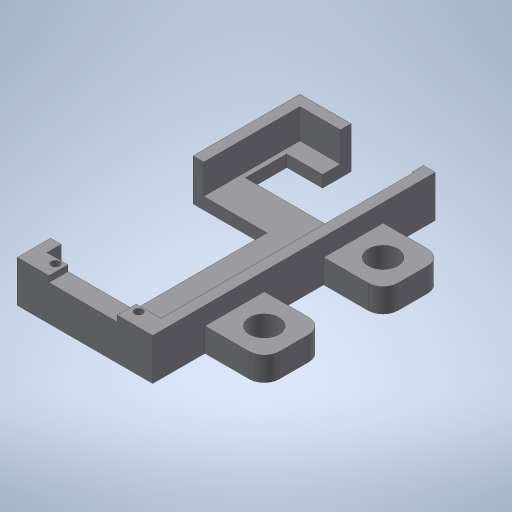
# Autodesk Inventor part: esp32-rev-tft-back-largeEncoderConn
Saved by Autodesk Inventor 2023.4 (Build 274418000, 418)
## iProperties
RuleStatus: InUse
Created: 2023-11-01
Part Number: esp32-rev-tft-back-largeEncoderConn
Project: COMMON
Material: Generic
Catalog Web Link: https://www.janelia.org/
Vendor: HHMI: JRC - jET
Document SubType Name: Modeling
Designer: sawtelles
Density: 1 g/cm^3
Appearance: Default
AfterDocSave0: file://Part Number Cleaner
LAB/DEPT: COMMON
REQUESTING SCIENTIST: COMMON
DESIGN DEPARTMENT: HHMI: JRC - jET
ALTERED ITEM PART NUMBER: N/A
ALTERED ITEM VENDOR: N/A
ALTERED ITEM DESCRIPTION: N/A
DocNumber: esp32-rev-tft=bezel
Folder: .
VDS_Category: Engineering
Title: Standard
Author: sawtelles
Revision Number: 0
Autodesk Inventor part; units mm, degrees
ref_plane "YZ Plane" through (0, 0, 0) normal (1, 0, 0) x (0, 1, 0)
ref_plane "XZ Plane" through (0, 0, 0) normal (0, 1, 0) x (-1, 0, 0)
ref_plane "XY Plane" through (0, 0, 0) normal (0, 0, 1) x (1, 0, 0)
sketch "Sketch1" plane through (0, 0, 0) normal (0, 1, 0) x (-1, 0, 0)
  line L0 (0, 0) -> (23.876, 0) construction
  line L1 (23.876, 0) -> (23.876, -71.882) construction
  line L2 (23.876, -71.882) -> (0, -71.882) construction
  line L3 (0, -71.882) -> (0, 0) construction
  line L4 (-0.254, 0.254) -> (24.13, 0.254)
  line L5 (24.13, 0.254) -> (24.13, -72.136)
  line L6 (24.13, -72.136) -> (-0.254, -72.136)
  line L7 (-0.254, -72.136) -> (-0.254, 0.254)
  circle A0 centre (5.2832, -21.971) radius 2.921
  circle A1 centre (12.2682, -21.971) radius 2.921
  circle A2 centre (19.2532, -21.971) radius 2.921
  circle A3 centre (12.2682, -58.801) radius 2.921
  circle A4 centre (21.1582, -16.891) radius 0.889
  circle A5 centre (3.3782, -16.891) radius 0.889
  circle A6 centre (21.8694, -62.611) radius 1.27
  circle A7 centre (2.7432, -62.611) radius 1.27
  line L8 (4.572, -26.416) -> (20.066, -26.416)
  line L9 (20.066, -26.416) -> (20.066, -53.848)
  line L10 (20.066, -53.848) -> (4.572, -53.848)
  line L11 (4.572, -53.848) -> (4.572, -26.416)
  dimension "d0" = 23.876
  dimension "d1" = 71.882
  dimension "d2" = 24.384
  dimension "d3" = 72.39
  dimension "d4" = 5.842
  dimension "d5" = 5.842
  dimension "d6" = 5.842
  dimension "d7" = 5.842
  dimension "d8" = 1.778
  dimension "d9" = 1.778
  dimension "d10" = 2.54
  dimension "d11" = 2.54
  dimension "d12" = 15.494
  dimension "d13" = 27.432
  dimension "d14" = 26.416
  constraints: 24 end point, 8 centre point, 6 parallel, 3 horizontal, 3 perpendicular
  measures "d0" distance of L1.end L2.end
  measures "d1" distance of L0.end L1.end
  measures "d2" distance of L5.end L6.end
  measures "d3" distance of L4.end L5.end
  measures "d4" diameter of A0
  measures "d5" diameter of A1
  measures "d6" diameter of A2
  measures "d7" diameter of A3
  measures "d8" diameter of A4
  measures "d9" diameter of A5
  measures "d10" diameter of A6
  measures "d11" diameter of A7
  measures "d12" distance of L9.end L10.end
  measures "d13" distance of L8.end L9.end
  measures "d14" distance from line of L0 L8.start
extrude "Extrusion1" add sketch "Sketch1" along normal blind 2.032
chamfer "Chamfer1" distance 0.762 angle 45 4 edges at (-16.3322, 2.032, -21.971) (-9.3472, 2.032, -21.971) (-2.3622, 2.032, -21.971) (-9.3472, 2.032, -58.801)
sketch "Sketch2" plane through (0, 0, 0) normal (0, -1, 0) x (1, 0, 0)
  line L0 (-24.13, -72.136) -> (-24.13, 0.254) projected
  line L1 (0.254, -72.136) -> (-24.13, -72.136)
  line L2 (-24.13, -72.136) -> (-24.13, -62.484)
  line L3 (-24.13, -62.484) -> (0.254, -62.484)
  line L4 (0.254, -62.484) -> (0.254, -72.136)
  line L5 (0.254, 0.254) -> (-24.13, 0.254)
  line L6 (-24.13, 0.254) -> (-24.13, -18.034)
  line L7 (-24.13, -18.034) -> (0.254, -18.034)
  line L8 (0.254, -18.034) -> (0.254, 0.254)
  circle A0 centre (-19.2532, -21.971) radius 2.921 projected
  circle A1 centre (-19.2532, -21.971) radius 2.54
  circle A2 centre (-12.1916, -21.971) radius 2.54
  circle A3 centre (-5.2239, -21.971) radius 2.54
  circle A4 centre (-12.2682, -58.801) radius 2.921 projected
  circle A5 centre (-12.2682, -58.801) radius 2.54
  point P0 (0, 0)
  point P1 (-24.13, 0.254)
  dimension "d20" = 9.652
  dimension "d21" = 18.288
  dimension "d26" = 5.08
  dimension "d27" = 5.08
  dimension "d28" = 5.08
  dimension "d29" = 5.08
  constraints: 16 end point, 4 centre point, 4 parallel, 2 coincident, 2 horizontal, 2 perpendicular, 2 point on line
  measures "d20" distance of L1.end L2.end
  measures "d21" distance of L6.end L5.end
  measures "d26" diameter of A1
  measures "d27" diameter of A2
  measures "d28" diameter of A3
  measures "d29" diameter of A5
extrude "Extrusion2" add sketch "Sketch2" along normal blind 2.032 contours L0 L3 L4 L1 | L0 L5 L8 L7
sketch "Sketch3" plane through (0, 2.032, 0) normal (0, 1, 0) x (1, 0, 0)
  circle A0 centre (-21.1582, 16.891) radius 0.889 projected
  circle A1 centre (-3.3782, 16.891) radius 0.889 projected
  circle A2 centre (-21.8694, 62.611) radius 1.27 projected
  circle A3 centre (-2.7432, 62.611) radius 1.27 projected
  point P0 (0, 0)
extrude "Extrusion3" cut sketch "Sketch3" against normal through all
sketch "Sketch4" plane through (0, 0, 0) normal (0, -1, 0) x (1, 0, 0)
  circle A0 centre (-19.2532, -21.971) radius 2.921 projected
  circle A1 centre (-19.2532, -21.971) radius 2.54
  circle A2 centre (-12.2682, -21.971) radius 2.921 projected
  circle A3 centre (-12.2682, -21.971) radius 2.54
  circle A4 centre (-5.2832, -21.971) radius 2.921 projected
  circle A5 centre (-5.2832, -21.971) radius 2.54
  circle A6 centre (-12.2682, -58.801) radius 2.921 projected
  circle A7 centre (-12.2682, -58.801) radius 2.54
  point P0 (0, 0)
  dimension "d30" = 5.08
  dimension "d31" = 5.08
  dimension "d32" = 5.08
  dimension "d33" = 5.08
  constraints: 4 centre point, 4 coincident
  measures "d30" diameter of A1
  measures "d31" diameter of A3
  measures "d32" diameter of A5
  measures "d33" diameter of A7
extrude "Extrusion4" [suppressed]
sketch "Sketch5" plane through (0, 0, 0) normal (0, -1, 0) x (1, 0, 0)
  line L0 (-24.13, -72.136) -> (-24.13, 0.254) projected
  line L1 (-24.13, -22.8093) -> (-19.2532, -22.8093)
  line L2 (-19.2532, -22.8093) -> (-19.2532, -21.1266)
  line L3 (-19.2532, -21.1266) -> (-24.13, -21.1266)
  line L4 (-24.13, -21.1266) -> (-24.13, -22.8093)
  line L5 (-15.5643, -22.8093) -> (-11.8565, -22.8093)
  line L6 (-11.8565, -22.8093) -> (-11.8565, -21.1266)
  line L7 (-11.8565, -21.1266) -> (-15.5643, -21.1266)
  line L8 (-15.5643, -21.1266) -> (-15.5643, -22.8093)
  line L9 (-8.5481, -22.8093) -> (-6.5231, -22.8093)
  line L10 (-6.5231, -22.8093) -> (-6.5231, -21.1266)
  line L11 (-6.5231, -21.1266) -> (-8.5481, -21.1266)
  line L12 (-8.5481, -21.1266) -> (-8.5481, -22.8093)
  line L13 (-16.1062, -59.6299) -> (-13.3967, -59.6299)
  line L14 (-13.3967, -59.6299) -> (-13.3967, -57.9472)
  line L15 (-13.3967, -57.9472) -> (-16.1062, -57.9472)
  line L16 (-16.1062, -57.9472) -> (-16.1062, -59.6299)
  point P0 (0, 0)
  constraints: 32 end point, 8 parallel, 5 point on line, 4 horizontal, 4 perpendicular
extrude "Extrusion5" [suppressed]
sketch "Sketch6" plane through (0, 2.032, 0) normal (0, 1, 0) x (1, 0, 0)
  line L0 (2.54, -2.54) -> (-26.416, -2.54)
  line L1 (-26.416, -2.54) -> (-26.416, 74.422)
  line L2 (-26.416, 74.422) -> (2.54, 74.422)
  line L3 (2.54, 74.422) -> (2.54, -2.54)
  line L4 (-24.13, 72.136) -> (-24.13, -0.254) projected
  line L5 (0.254, 72.136) -> (-24.13, 72.136) projected
  line L6 (-24.13, -0.254) -> (0.254, -0.254) projected
  line L7 (0.254, -0.254) -> (0.254, 72.136) projected
  point P0 (0, 0)
  dimension "d38" = 2.286
  dimension "d39" = 2.286
  constraints: 8 end point, 2 parallel, 1 horizontal, 1 perpendicular
  measures "d38" distance between parallel lines of L1 L4
  measures "d39" distance between parallel lines of L2 L5
extrude "Extrusion6" add sketch "Sketch6" against normal blind 13.462
sketch "Sketch7" plane through (0, -11.43, 0) normal (0, -1, 0) x (1, 0, 0)
  line L0 (-5.334, -1.381) -> (-18.542, -1.381)
  line L1 (-18.542, -1.381) -> (-18.542, 4.3401)
  line L2 (-18.542, 4.3401) -> (-5.334, 4.3401)
  line L3 (-5.334, 4.3401) -> (-5.334, -1.381)
  line L4 (-5.334, -1.381) -> (-18.542, 4.3401) construction
  line L5 (-18.542, -1.381) -> (-5.334, 4.3401) construction
  point P0 (0, 0)
  point P1 (-11.938, 1.4796)
  dimension "d42" = 13.208
  constraints: 12 end point, 2 midpoint, 2 parallel, 1 horizontal, 1 perpendicular
  measures "d42" distance of L1.end L2.end
extrude "Extrusion7" [suppressed]
sketch "Sketch8" plane through (0, -2.032, 0) normal (0, -1, 0) x (1, 0, 0)
  line L0 (0.254, -18.034) -> (0.254, 0.254) projected
  line L1 (0.254, 0.254) -> (-2.921, 0.254)
  line L2 (-2.921, 0.254) -> (-2.921, -2.921)
  line L3 (-2.921, -2.921) -> (0.254, -2.921)
  line L4 (0.254, -2.921) -> (0.254, 0.254)
  line L5 (-24.13, 0.254) -> (-24.13, -18.034) projected
  line L6 (-24.13, 0.254) -> (-20.955, 0.254)
  line L7 (-20.955, 0.254) -> (-20.955, -2.921)
  line L8 (-20.955, -2.921) -> (-24.13, -2.921)
  line L9 (-24.13, -2.921) -> (-24.13, 0.254)
  line L10 (-24.13, -62.484) -> (-24.13, -72.136) projected
  line L11 (-24.13, -72.136) -> (-20.955, -72.136)
  line L12 (-20.955, -72.136) -> (-20.955, -68.961)
  line L13 (-20.955, -68.961) -> (-24.13, -68.961)
  line L14 (-24.13, -68.961) -> (-24.13, -72.136)
  line L15 (0.254, -72.136) -> (0.254, -62.484) projected
  line L16 (0.254, -72.136) -> (-2.921, -72.136)
  line L17 (-2.921, -72.136) -> (-2.921, -68.961)
  line L18 (-2.921, -68.961) -> (0.254, -68.961)
  line L19 (0.254, -68.961) -> (0.254, -72.136)
  point P0 (0, 0)
  point P1 (0.254, -68.961)
  dimension "d45" = 3.175
  dimension "d46" = 3.175
  dimension "d47" = 3.175
  dimension "d48" = 3.175
  dimension "d49" = 3.175
  dimension "d50" = 3.175
  dimension "d51" = 3.175
  dimension "d52" = 3.175
  constraints: 32 end point, 8 parallel, 4 horizontal, 4 perpendicular
  measures "d45" distance of L3.end L2.end
  measures "d46" distance of L2.end L1.end
  measures "d47" distance of L7.end L8.end
  measures "d48" distance of L6.end L7.end
  measures "d49" distance of L13.end L12.end
  measures "d50" distance of L12.end L11.end
  measures "d51" distance of L17.end L18.end
  measures "d52" distance of L16.end L17.end
extrude "Extrusion8" [suppressed]
chamfer "Chamfer2" [suppressed]
chamfer "Chamfer3" [suppressed]
sketch "Sketch9" plane through (0, -11.43, 0) normal (0, -1, 0) x (1, 0, 0)
  line L0 (2.54, -74.422) -> (2.54, 2.54) projected
  line L1 (2.54, -13.97) -> (-28.1751, -13.97)
  line L2 (-28.1751, -13.97) -> (-28.1751, 11.3497)
  line L3 (-28.1751, 11.3497) -> (2.54, 11.3497)
  line L4 (2.54, 11.3497) -> (2.54, -13.97)
  point P0 (0, 0)
  constraints: 8 end point, 2 parallel, 1 horizontal, 1 perpendicular, 1 point on line
extrude "Extrusion9" cut sketch "Sketch9" against normal blind 25.4
sketch "Sketch10" plane through (0, -2.032, 0) normal (0, -1, 0) x (1, 0, 0)
  line L0 (-24.13, -18.034) -> (0.254, -18.034) projected
  line L1 (-24.13, -18.034) -> (0.254, -18.034) projected
  circle A0 centre (-3.3782, -16.891) radius 0.889 projected
  line L2 (0.254, -13.97) -> (-24.13, -13.97) projected
  circle A1 centre (-21.1582, -16.891) radius 0.889 projected
  line L3 (-24.13, -18.034) -> (0.254, -18.034) projected
  line L4 (-24.13, -13.97) -> (-24.13, -18.034) projected
  line L5 (0.254, -18.034) -> (0.254, -13.97) projected
  point P0 (0, 0)
  point P1 (-2.8246, -18.034)
  point P2 (-20.6046, -18.034)
  point P3 (-3.9318, -18.034)
  point P4 (-21.7118, -18.034)
  constraints: 2 other
extrude "Extrusion10" add sketch "Sketch10" along normal blind 9.398
sketch "Sketch12" plane through (0, -11.43, 0) normal (0, -1, 0) x (1, 0, 0)
  line L0 (0.254, -18.034) -> (-24.13, -18.034) projected
  line L1 (-24.13, -72.136) -> (-24.13, -18.034) projected
  line L2 (0.254, -18.034) -> (-24.13, -18.034)
  line L3 (-24.13, -18.034) -> (-24.13, -72.136)
  line L4 (-24.13, -72.136) -> (0.254, -72.136)
  line L5 (0.254, -72.136) -> (0.254, -18.034)
  point P0 (0, 0)
  point P1 (-2.8246, -18.034)
  point P2 (-2.8246, -18.034)
  point P3 (-24.13, -18.034)
  constraints: 8 end point, 2 parallel, 1 horizontal, 1 perpendicular
extrude "Extrusion11" add sketch "Sketch12" against normal blind 2.54
sketch "Sketch13" plane through (0, 2.032, 0) normal (0, 1, 0) x (1, 0, 0)
  circle A0 centre (-2.7432, 62.611) radius 1.27 projected
  circle A1 centre (-21.8694, 62.611) radius 1.27 projected
  point P0 (0, 0)
extrude "Extrusion12" [suppressed]
sketch "Sketch15" plane through (2.54, 2.032, -74.422) normal (0, 0, -1) x (-1, 0, 0)
  line L0 (0, 0) -> (28.956, 0) projected
  line L1 (0, 0) -> (30.6199, 0)
  line L2 (30.6199, 0) -> (30.6199, -4.572)
  line L3 (30.6199, -4.572) -> (0, -4.572)
  line L4 (0, -4.572) -> (0, 0)
  point P0 (2.54, -2.032)
  dimension "d70" = 4.572
  constraints: 8 end point, 2 parallel, 1 horizontal, 1 perpendicular
  measures "d70" distance of L1.end L2.end
extrude "Extrusion13" cut sketch "Sketch15" against normal through all
sketch "Sketch18" plane through (0, -11.43, 0) normal (0, -1, 0) x (1, 0, 0)
  line L0 (-23.114, -68.326) -> (-15.494, -68.326)
  line L1 (-15.494, -68.326) -> (-15.494, -59.436)
  line L2 (-15.494, -59.436) -> (-23.114, -59.436)
  line L3 (-23.114, -59.436) -> (-23.114, -68.326)
  line L4 (-26.416, -13.97) -> (-26.416, -74.422) projected
  line L5 (-26.416, -51.562) -> (-10.5664, -51.562)
  line L6 (-10.5664, -51.562) -> (-10.5664, -21.082)
  line L7 (-10.5664, -21.082) -> (-26.416, -21.082)
  line L8 (-26.416, -21.082) -> (-26.416, -51.562)
  point P0 (0, 0)
  dimension "d73" = 7.62
  dimension "d74" = 8.89
  dimension "d75" = 15.8496
  dimension "d76" = 30.48
  dimension "d95" = 3.302
  constraints: 16 end point, 4 parallel, 2 horizontal, 2 perpendicular, 1 point on line
  measures "d73" distance of L2.end L1.end
  measures "d74" distance of L1.end L0.end
  measures "d75" distance of L7.end L6.end
  measures "d76" distance of L6.end L5.end
  measures "d95" distance between parallel lines of L4 L3
extrude "Extrusion14" cut sketch "Sketch18" against normal through all
sketch "Sketch20" plane through (-26.416, -2.54, -74.422) normal (0, 1, 0) x (1, 0, 0)
  line L0 (28.956, -60.452) -> (0, -60.452) projected
  line L1 (6.7783, -60.452) -> (21.3663, -60.452)
  line L2 (21.3663, -60.452) -> (21.3663, -55.9866)
  line L3 (21.3663, -55.9866) -> (6.7783, -55.9866)
  line L4 (6.7783, -55.9866) -> (6.7783, -60.452)
  point P0 (26.416, -74.422)
  constraints: 8 end point, 2 parallel, 1 horizontal, 1 perpendicular, 1 point on line
extrude "Extrusion15" cut sketch "Sketch20" against normal blind 1.27
sketch "Sketch22" plane through (-26.416, -2.54, -74.422) normal (0, 1, 0) x (1, 0, 0)
  line L0 (2.286, -2.286) -> (26.67, -2.286) projected
  line L1 (14.0723, -2.286) -> (23.0495, -2.286)
  line L2 (23.0495, -2.286) -> (23.0495, 1.6439)
  line L3 (23.0495, 1.6439) -> (14.0723, 1.6439)
  line L4 (14.0723, 1.6439) -> (14.0723, -2.286)
  point P0 (26.416, -74.422)
  point P1 (23.0495, -2.286)
  constraints: 8 end point, 2 parallel, 1 horizontal, 1 perpendicular, 1 point on line
extrude "Extrusion16" cut sketch "Sketch22" against normal blind 4.318
sketch "Sketch23" plane through (2.54, -11.43, -13.97) normal (1, 0, 0) x (0, 0, -1)
  line L0 (60.452, 0) -> (0, 0) projected
  line L1 (11.176, 0) -> (23.876, 0)
  line L2 (23.876, 0) -> (23.876, 5.08)
  line L3 (23.876, 5.08) -> (11.176, 5.08)
  line L4 (11.176, 5.08) -> (11.176, 0)
  line L5 (36.576, 0) -> (49.276, 0)
  line L6 (49.276, 0) -> (49.276, 5.08)
  line L7 (49.276, 5.08) -> (36.576, 5.08)
  line L8 (36.576, 5.08) -> (36.576, 0)
  point P0 (-13.97, 11.43)
  dimension "d83" = 12.7
  dimension "d84" = 5.08
  dimension "d85" = 12.7
  constraints: 16 end point, 4 parallel, 2 horizontal, 2 perpendicular, 2 point on line
  measures "d83" distance of L3.end L2.end
  measures "d84" distance of L2.end L1.end
  measures "d85" distance of L7.end L6.end
extrude "Extrusion17" add sketch "Sketch23" along normal blind 12.7
sketch "Sketch24" plane through (2.54, -6.35, -25.146) normal (0, 1, 0) x (1, 0, 0)
  circle A0 centre (6.35, 6.35) radius 3.175
  circle A1 centre (6.35, 31.75) radius 3.175
  point P0 (-2.54, -25.146)
  dimension "d88" = 6.35
  dimension "d89" = 6.35
  constraints: 2 centre point
  measures "d88" diameter of A0
  measures "d89" diameter of A1
extrude "Extrusion18" cut sketch "Sketch24" against normal through all
fillet "Fillet1" radius 3.175 4 edges at (15.24, -8.89, -37.846) (15.24, -8.89, -50.546) (15.24, -8.89, -63.246) (15.24, -8.89, -25.146)
sketch "Sketch25" plane through (0, -11.43, 0) normal (0, -1, 0) x (1, 0, 0)
  line L0 (-20.1426, -70.0681) -> (-13.3239, -70.0681) construction
  line L1 (-13.3239, -70.0681) -> (-13.3239, -72.6545) construction
  line L2 (-13.3239, -72.6545) -> (-20.1426, -72.6545) construction
  line L3 (-20.1426, -72.6545) -> (-20.1426, -70.0681) construction
  line L4 (-10.475, -22.5499) -> (-4.7735, -22.5499) construction
  line L5 (-4.7735, -22.5499) -> (-4.7735, -37.4146) construction
  line L6 (-4.7735, -37.4146) -> (-10.475, -37.4146) construction
  line L7 (-10.475, -37.4146) -> (-10.475, -22.5499) construction
  line L8 (-18.1938, -73.1804) -> (-19.6807, -73.1804)
  line L9 (-19.6807, -73.1804) -> (-19.6807, -72.8691)
  line L10 (-19.6807, -72.8691) -> (-19.1275, -72.8691)
  line L11 (-19.1275, -72.8691) -> (-19.1275, -70.8264)
  line L12 (-19.1275, -70.8264) -> (-19.6807, -70.8264)
  line L13 (-19.6807, -70.8264) -> (-19.6807, -70.5473)
  spline S0 degree 2 poles (-19.6807, -70.5473) (-19.367, -70.5473) (-19.0706, -70.3695) (-19.0509, -70.1225) knots 0 0 0 1 2 2 2
  line L14 (-19.0509, -70.1225) -> (-18.7347, -70.1225)
  line L15 (-18.7347, -70.1225) -> (-18.7347, -72.8691)
  line L16 (-18.7347, -72.8691) -> (-18.1938, -72.8691)
  line L17 (-18.1938, -72.8691) -> (-18.1938, -73.1804)
  line L18 (-13.1352, -73.1804) -> (-15.0149, -73.1804)
  line L19 (-15.0149, -73.1804) -> (-15.0149, -72.7481)
  spline S1 degree 2 poles (-15.0149, -72.7481) (-14.8123, -72.5579) (-14.4517, -72.2047) (-14.2788, -72.0145) knots 0 0 0 1 2 2 2
  spline S2 degree 2 poles (-14.2788, -72.0145) (-13.9305, -71.6317) (-13.6761, -71.1722) (-13.6761, -70.9277) knots 0 0 0 1 2 2 2
  spline S3 degree 2 poles (-13.6761, -70.9277) (-13.6761, -70.7993) (-13.7552, -70.6066) (-13.8268, -70.5449) knots 0 0 0 1 2 2 2
  spline S4 degree 2 poles (-13.8268, -70.5449) (-13.8984, -70.4831) (-14.0862, -70.4213) (-14.1998, -70.4213) knots 0 0 0 1 2 2 2
  spline S5 degree 2 poles (-14.1998, -70.4213) (-14.3085, -70.4213) (-14.5308, -70.4757) (-14.632, -70.5177) knots 0 0 0 1 2 2 2
  spline S6 degree 2 poles (-14.632, -70.5177) (-14.7185, -70.5523) (-14.879, -70.6511) (-14.9284, -70.6856) knots 0 0 0 1 2 2 2
  line L20 (-14.9284, -70.6856) -> (-14.9507, -70.6856)
  line L21 (-14.9507, -70.6856) -> (-14.9507, -70.2509)
  spline S7 degree 2 poles (-14.9507, -70.2509) (-14.8247, -70.1892) (-14.3727, -70.0681) (-14.1701, -70.0681) knots 0 0 0 1 2 2 2
  spline S8 degree 2 poles (-14.1701, -70.0681) (-13.7428, -70.0681) (-13.2612, -70.5202) (-13.2612, -70.9055) knots 0 0 0 1 2 2 2
  spline S9 degree 2 poles (-13.2612, -70.9055) (-13.2612, -71.0858) (-13.3451, -71.3871) (-13.4192, -71.5156) knots 0 0 0 1 2 2 2
  spline S10 degree 2 poles (-13.4192, -71.5156) (-13.4933, -71.6489) (-13.7082, -71.9108) (-13.8268, -72.0367) knots 0 0 0 1 2 2 2
  spline S11 degree 2 poles (-13.8268, -72.0367) (-14.0195, -72.2467) (-14.4912, -72.6962) (-14.632, -72.8271) knots 0 0 0 1 2 2 2
  line L22 (-14.632, -72.8271) -> (-13.1352, -72.8271)
  line L23 (-13.1352, -72.8271) -> (-13.1352, -73.1804)
  point P0 (0, 0)
  constraints: 4 other
extrude "Extrusion19" cut sketch "Sketch25" against normal blind 0.127
sketch "Sketch26" plane through (0, -8.89, 0) normal (0, 1, 0) x (1, 0, 0)
  line L0 (-15.494, 68.326) -> (-15.494, 59.436) projected
  line L1 (-15.494, 59.436) -> (0, 59.436)
  line L2 (0, 59.436) -> (0, 80.1372)
  line L3 (0, 80.1372) -> (-15.494, 80.1372)
  line L4 (-15.494, 80.1372) -> (-15.494, 59.436)
  point P0 (0, 0)
  constraints: 8 end point, 2 parallel, 1 horizontal, 1 perpendicular
extrude "Extrusion20" cut sketch "Sketch26" along normal mid plane 25.4
sketch "Sketch27" plane through (0, -8.89, 0) normal (0, 1, 0) x (1, 0, 0)
  line L0 (0.254, 72.136) -> (0.254, 18.034) projected
  line L1 (0.254, 18.034) -> (-5.1408, 18.034)
  line L2 (-5.1408, 18.034) -> (-5.1408, 18.7364)
  line L3 (-5.1408, 18.7364) -> (0.254, 18.7364)
  line L4 (0.254, 18.7364) -> (0.254, 18.034)
  line L5 (-24.13, 18.034) -> (-19.4345, 18.034)
  line L6 (-19.4345, 18.034) -> (-19.4345, 18.7364)
  line L7 (-19.4345, 18.7364) -> (-24.13, 18.7364)
  line L8 (-24.13, 18.7364) -> (-24.13, 18.034)
  point P0 (0, 0)
  constraints: 16 end point, 4 parallel, 2 horizontal, 2 perpendicular, 1 point on line
extrude "Extrusion21" [suppressed]
body "Solid1"
